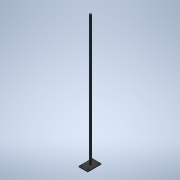
# Autodesk Inventor part: rotatable rod table
Saved by Autodesk Inventor 2020 (Build 240168000, 168)
## iProperties
Created: 2015-02-10
Part Number: rotatable rod table
Material: Generic
Document SubType Name: Modeling
Designer: Pascal
Density: 1 g/cm^3
Appearance: Generic
Mass: 12.4916 g
Surface Area: 85.0197 cm^2
Volume: 12.4916 cm^3
Author: Pascal
Autodesk Inventor part; units mm, degrees
ref_plane "YZ Plane" through (0, 0, 0) normal (1, 0, 0) x (0, 1, 0)
ref_plane "XZ Plane" through (0, 0, 0) normal (0, 1, 0) x (-1, 0, 0)
ref_plane "XY Plane" through (0, 0, 0) normal (0, 0, 1) x (1, 0, 0)
sketch "Sketch1" plane through (0, 0, 0) normal (0, 1, 0) x (-1, 0, 0)
  line L0 (13.2677, 19.6408) -> (-12.1323, 19.6408)
  line L1 (-12.1323, 19.6408) -> (-12.1323, -18.4592)
  line L2 (-12.1323, -18.4592) -> (13.2677, -18.4592)
  line L3 (13.2677, -18.4592) -> (13.2677, 19.6408)
  point P0 (0, 0)
  dimension "d0" = 25.4
  dimension "d1" = 38.1
  constraints: 8 end point, 2 parallel, 1 horizontal, 1 perpendicular
  measures "d0" distance of L1.end L2.end
  measures "d1" distance of L2.end L0.start
extrude "Extrusion1" add sketch "Sketch1" along normal blind 3.175
hole "Hole1" at (-9.6799, 3.175, 14.8783) direction (0, -1, 0) diameter 4.4958 depth 3.175 clearance for "Flat Head Machine Screw (82)" size "#8" standard "Ansi Unified Screw Threads"
hole "Hole2" at (8.5446, 3.175, 14.8783) direction (0, -1, 0) diameter 4.4958 depth 3.175 clearance for "Flat Head Machine Screw (82)" size "#8" standard "Ansi Unified Screw Threads"
hole "Hole3" at (-9.6799, 3.175, -13.6967) direction (0, -1, 0) diameter 4.4958 depth 3.175 clearance for "Flat Head Machine Screw (82)" size "#8" standard "Ansi Unified Screw Threads"
hole "Hole4" at (8.5446, 3.175, -13.6967) direction (0, -1, 0) diameter 4.4958 depth 3.175 clearance for "Flat Head Machine Screw (82)" size "#8" standard "Ansi Unified Screw Threads"
sketch "Sketch2" plane through (0, 3.175, 0) normal (0, 1, 0) x (1, 0, 0)
  circle A0 centre (0, 0) radius 3.175
  dimension "d58" = 6.35
  constraints: 1 centre point, 1 coincident
  measures "d58" diameter of A0
extrude "Extrusion2" add sketch "Sketch2" along normal blind 304.8
sketch "Sketch3" plane through (0, 0, 0) normal (1, 0, 0) x (0, 1, 0)
  point P0 (0, 0)
sketch "Sketch4" plane through (0, 307.975, 0) normal (0, 1, 0) x (1, 0, 0)
  circle A0 centre (0, 0) radius 3.175 projected
extrude "Extrusion3" add sketch "Sketch4" along normal blind 63.5
body "Solid1"
